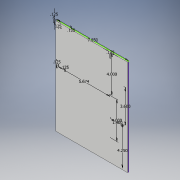
# Autodesk Inventor part: ElectronicsPlate
Saved by Autodesk Inventor 2017 (Build 210142000, 142)
## iProperties
Created: 2018-01-06
Part Number: ElectronicsPlate
Material: Generic
Document SubType Name: Modeling
Designer: User
Density: 1 g/cm^3
Appearance: Default
Author: User
Autodesk Inventor part; units mm, degrees
ref_plane "YZ Plane" through (0, 0, 0) normal (1, 0, 0) x (0, 1, 0)
ref_plane "XZ Plane" through (0, 0, 0) normal (0, 1, 0) x (-1, 0, 0)
ref_plane "XY Plane" through (0, 0, 0) normal (0, 0, 1) x (1, 0, 0)
sketch "Sketch1" plane through (0, 0, 0) normal (0, 0, 1) x (1, 0, 0)
  line L0 (0, 0) -> (199.39, 0)
  line L1 (199.39, 0) -> (199.39, 266.7)
  line L2 (199.39, 266.7) -> (0, 266.7)
  line L3 (0, 266.7) -> (0, 0)
  line L4 (12.1493, 266.7) -> (12.1493, 263.525)
  line L5 (0, 247.1772) -> (3.175, 247.1772)
  line L6 (3.175, 263.525) -> (147.2946, 263.525)
  line L7 (147.2946, 263.525) -> (147.2946, 161.925)
  line L8 (147.2946, 161.925) -> (3.175, 161.925)
  line L9 (3.175, 161.925) -> (3.175, 263.525)
  line L10 (5.8968, 161.925) -> (5.8968, 158.75)
  line L11 (3.175, 158.75) -> (147.2946, 158.75)
  line L12 (147.2946, 158.75) -> (147.2946, 57.15)
  line L13 (147.2946, 57.15) -> (3.175, 57.15)
  line L14 (3.175, 57.15) -> (3.175, 158.75)
  line L15 (147.2946, 247.6224) -> (150.4696, 247.6224)
  line L16 (150.4696, 199.39) -> (186.0296, 199.39)
  line L17 (186.0296, 199.39) -> (186.0296, 107.95)
  line L18 (186.0296, 107.95) -> (150.4696, 107.95)
  line L19 (150.4696, 107.95) -> (150.4696, 199.39)
  dimension "d0" = 199.39
  dimension "d2" = 3.175
  dimension "d3" = 3.175
  dimension "d4" = 144.1196
  dimension "d5" = 101.6
  dimension "d6" = 3.175
  dimension "d7" = 101.6
  dimension "d8" = 3.175
  dimension "d9" = 35.56
  dimension "d10" = 91.44
  dimension "d11" = 107.95
  dimension "d12" = 3.175
  dimension "d13" = 3.175
  constraints: 40 end point, 8 parallel, 7 perpendicular, 5 horizontal, 4 point on line
  measures "d0" distance of L2.end L1.end
  measures "d2" distance of L4.start L4.end
  measures "d3" distance of L5.start L5.end
  measures "d4" distance of L7.end L8.end
  measures "d5" distance of L6.end L7.end
  measures "d6" distance of L10.start L10.end
  measures "d7" distance of L11.end L12.end
  measures "d8" distance of L15.start L15.end
  measures "d9" distance of L17.end L18.end
  measures "d10" distance of L16.end L17.end
  measures "d11" distance between parallel lines of L0 L18
  measures "d12" distance between parallel lines of L2 L6
  measures "d13" distance between parallel lines of L8 L11
sketch "Sketch2" plane through (0, 0, 0) normal (0, 0, 1) x (1, 0, 0)
  line L0 (199.39, 0) -> (0, 0)
  line L1 (0, 0) -> (0, 266.7)
  line L2 (0, 266.7) -> (199.39, 266.7)
  line L3 (199.39, 266.7) -> (199.39, 0)
  point P0 (0, 0)
  constraints: 8 end point, 2 parallel, 1 horizontal, 1 perpendicular
extrude "Extrusion1" add sketch "Sketch2" along normal blind 3.175
body "Solid1"
